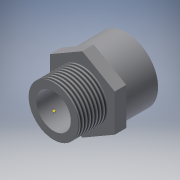
# Autodesk Inventor part: PVCConnectorMale3_4inch
Saved by Autodesk Inventor 2016 (Build 200138000, 138)
## iProperties
Created: 2015-11-20
Part Number: PVCConnectorMale3_4inch
Material: Generic
Document SubType Name: Modeling
Designer: al11g09
Density: 1 g/cm^3
Appearance: Default
Author: al11g09
Autodesk Inventor part; units mm, degrees
ref_plane "YZ Plane" through (0, 0, 0) normal (1, 0, 0) x (0, 1, 0)
ref_plane "XZ Plane" through (0, 0, 0) normal (0, 1, 0) x (-1, 0, 0)
ref_plane "XY Plane" through (0, 0, 0) normal (0, 0, 1) x (1, 0, 0)
sketch "Sketch1" plane through (0, 0, 0) normal (0, 1, 0) x (-1, 0, 0)
  circle A0 centre (0, 0) radius 13.5
  circle A1 centre (0, 0) radius 16.5
  dimension "d0" = 27
  dimension "d1" = 33
  constraints: 2 centre point, 2 coincident
  measures "d0" diameter of A0
  measures "d1" diameter of A1
extrude "pipeEnd" add sketch "Sketch1" along normal blind 17
sketch "Sketch2" plane through (0, 0, 0) normal (0, 1, 0) x (-1, 0, 0)
  circle A0 centre (0, 0) radius 19.5 construction
  line L0 (16.8875, -9.75) -> (16.8875, 9.75)
  line L1 (16.8875, 9.75) -> (0, 19.5)
  line L2 (0, 19.5) -> (-16.8875, 9.75)
  line L3 (-16.8875, 9.75) -> (-16.8875, -9.75)
  line L4 (-16.8875, -9.75) -> (0, -19.5)
  line L5 (0, -19.5) -> (16.8875, -9.75)
  circle A1 centre (0, 0) radius 11
  dimension "d4" = 39
  dimension "d12" = 22
  constraints: 12 end point, 6 point on circle, 4 equal length, 2 centre point, 2 coincident, 2 vertical
  measures "d4" diameter of A0
  measures "d12" diameter of A1
extrude "hexBit" add sketch "Sketch2" against normal blind 6
sketch "Sketch3" plane through (0, -6, 0) normal (0, -1, 0) x (1, 0, 0)
  circle A0 centre (0, 0) radius 9
  circle A1 centre (0, 0) radius 13
  dimension "d7" = 18
  dimension "d8" = 26
  constraints: 2 centre point, 2 coincident
  measures "d7" diameter of A0
  measures "d8" diameter of A1
extrude "thread" add sketch "Sketch3" along normal blind 15
thread "Thread1" size "G 3/4-14" class "A" standard "BSP Pipe Threads" full length
sketch "pinsPlacement" plane through (0, -21, 0) normal (0, -1, 0) x (1, 0, 0)
  point P0 (0, 0)
  point P1 (0, 0)
  constraints: 1 coincident
body "Solid1"
